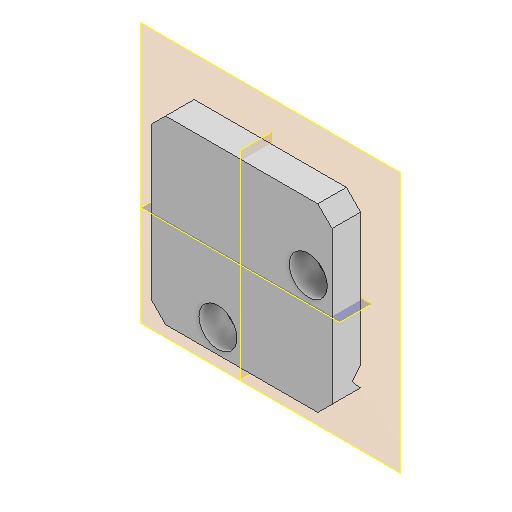
# Autodesk Inventor part: 20_Cube_Insert_Kinematic_Astromedia_30x40x1_45_pro_magnetic
Saved by Autodesk Inventor 2022 (Build 260153000, 153)
## iProperties
Created: 2021-11-15
Part Number: 20_Cube_Insert_Kinematic_Astromedia_30x40x1_45_pro_magnetic
Material: Generic
Document SubType Name: Modeling
Designer: diederichbenedict
Density: 1 g/cm^3
Appearance: Default
Catalog Web Link: isPrinted
Vendor: openUC2
Author: diederichbenedict
Autodesk Inventor part; units mm, degrees
ref_plane "YZ Plane" through (0, 0, 0) normal (1, 0, 0) x (0, 1, 0)
ref_plane "XZ Plane" through (0, 0, 0) normal (0, 1, 0) x (-1, 0, 0)
ref_plane "XY Plane" through (0, 0, 0) normal (0, 0, 1) x (1, 0, 0)
ref_plane "Work Plane1" through (0, 0, 2) normal (0, 0, 1) x (1, 0, 0)
sketch "Sketch1" plane through (0, 0, 2) normal (0, 0, 1) x (1, 0, 0)
  line L0 (-37.0712, 14) -> (-9.0712, 14) construction
  line L1 (-9.0712, 14) -> (-9.0712, -14) construction
  line L2 (-9.0712, -14) -> (-37.0712, -14) construction
  line L3 (-37.0712, -14) -> (-37.0712, 14) construction
  line L4 (-4.0712, -19) -> (-4.0712, 19)
  line L5 (-4.0712, 19) -> (-42.0712, 19)
  line L6 (-42.0712, 19) -> (-42.0712, -19)
  line L7 (-42.0712, -19) -> (-4.0712, -19)
  circle A0 centre (-23.0712, 0) radius 12.8
  point P0 (0, 0)
  dimension "d0" = 5
  constraints: 16 end point, 4 parallel, 2 perpendicular, 1 centre point, 1 horizontal, 3 other
  measures "d0" distance between parallel lines of L1 L4
extrude "Extrusion1" add sketch "Sketch1" along normal blind 6 contours L7 L6 L5 L4 | A0
sketch "Sketch3" plane through (0, 0, 2) normal (0, 0, -1) x (-1, 0, 0)
  circle A0 centre (9.0712, -14) radius 1.45 construction
  circle A1 centre (9.0712, -14) radius 2.45
  circle A2 centre (37.0712, -14) radius 1.45 projected
  circle A3 centre (37.0712, -14) radius 1.95
  point P0 (0, 0)
  dimension "d8" = 1
  dimension "d10" = 0.5
  constraints: 2 centre point
  measures "d8" radial gap between concentric circles of A0 A1
  measures "d10" radial gap between concentric circles of A2 A3
chamfer "Chamfer1" distance 3 angle 45 4 edges at (-42.0712, 19, 5) (-4.0712, 19, 5) (-4.0712, -19, 5) (-42.0712, -19, 5)
hole "Hole1" at (-37.0712, -14, 2) direction (0, 0, 1) diameter 4 depth 0.1 tip angle 100
sketch "Sketch4" plane through (-4.0712, -19, 2) normal (1, 0, 0) x (0, 0, -1)
  line L0 (2, 4.45) -> (6, 4.45)
  line L1 (2, 1.55) -> (6, 1.55)
  line L2 (0, 0) -> (0, 38) projected
  arc A0 (2, 19) -> (2, 19) centre (1.5, 4.4206) ccw projected
  line L3 (-1.7782, 5) -> (-0.1, 7) projected
  line L4 (-1.7782, 5) -> (-0.1, 3) projected
  line L5 (-0.1, 7) -> (0.6045, 7)
  line L6 (0.6045, 7) -> (0.6045, 3)
  line L7 (0.6045, 3) -> (-0.1, 3)
  line L8 (-0.1, 3) -> (-0.1, 7)
  constraints: 12 end point, 3 horizontal, 2 parallel, 1 perpendicular, 4 other
extrude "Extrusion4" cut sketch "Sketch4" against normal blind 8 contours L7 L8 L5 L2 | L2 L5 L6 L7 | L4 L3 L8
ref_plane "Arbeitsebene2" through (-23.0712, -12, 2) normal (1, 0, 0) x (0, 0, -1)
ref_plane "Arbeitsebene3" through (-39.0712, 0, 2) normal (0, -1, 0) x (1, 0, 0)
sketch "Skizze9" plane through (0, 0, 2) normal (0, 0, -1) x (-1, 0, 0)
  line L0 (12.0712, -16) -> (4.0712, -16) projected
  line L1 (7.0712, -19) -> (4.0712, -16) projected
  line L2 (39.0712, -19) -> (7.0712, -19) projected
  line L3 (42.0712, -16) -> (39.0712, -19) projected
  line L4 (42.0712, 16) -> (42.0712, -16) projected
  line L5 (39.0712, 19) -> (42.0712, 16) projected
  line L6 (7.0712, 19) -> (39.0712, 19) projected
  line L7 (4.0712, 16) -> (7.0712, 19) projected
  line L8 (4.0712, -12) -> (4.0712, 16) projected
  line L9 (4.0712, -12) -> (12.0712, -12) projected
  line L10 (12.0712, -12) -> (12.0712, -16) projected
  circle A0 centre (37.0712, -14) radius 2 projected
  circle A1 centre (28.0712, -14) radius 3
  circle A2 centre (9.0712, 5) radius 3
  point P0 (0, 0)
  dimension "d54" = 6
  dimension "d55" = 6
  dimension "d56" = 14
  dimension "d57" = 5
  dimension "d58" = 5
  dimension "d59" = 14
  constraints: 2 centre point
  measures "d54" diameter of A1
  measures "d55" diameter of A2
  measures "d56" distance from line of L4 A1.centre
  measures "d57" distance from line of A1.centre L2
  measures "d58" distance from line of L8 A2.centre
  measures "d59" distance from line of L6 A2.centre
extrude "Extrusion9" cut sketch "Skizze9" against normal blind 3 draft -2 contours A1 | A2
sketch "Skizze10" plane through (0, 0, 8) normal (0, 0, 1) x (1, 0, 0)
  circle A0 centre (-9.0712, 5) radius 4.05 projected
  circle A1 centre (-28.0712, -14) radius 4.55 projected
  circle A2 centre (-9.0712, 5) radius 4
  circle A3 centre (-28.0712, -14) radius 2.8952 projected
  circle A4 centre (-28.0712, -14) radius 4
  point P0 (0, 0)
  dimension "d62" = 8
  dimension "d63" = 8
  constraints: 2 centre point, 2 coincident
  measures "d62" diameter of A2
  measures "d63" diameter of A4
extrude "Extrusion10" cut sketch "Skizze10" against normal blind 5.5 contours A2 | A3 | A4
equation "\"d54\" = d55"
equation "\"d59\" = d56"
body "Solid1"
